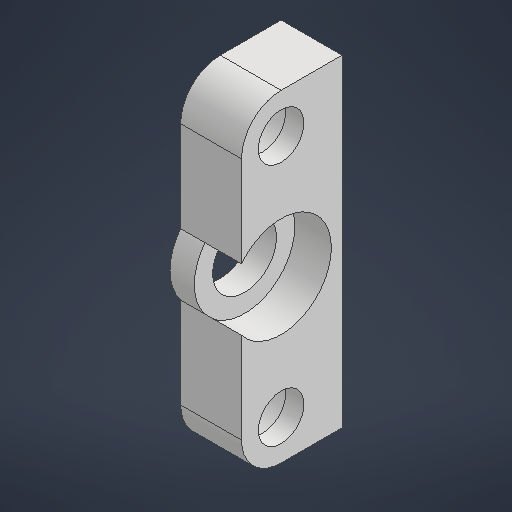
# Autodesk Inventor part: PCB_Housing_07_V4
Saved by Autodesk Inventor 2026.2 (Build 302298000, 298)
## iProperties
Created: 2026-03-17
Part Number: PCB_Housing_07_V4
Material: Generic
Document SubType Name: Modeling
Designer: vckot
Density: 1 g/cm^3
Appearance: Default
Author: vckot
Autodesk Inventor part; units mm, degrees
ref_plane "YZ Plane" through (0, 0, 0) normal (1, 0, 0) x (0, 1, 0)
ref_plane "XZ Plane" through (0, 0, 0) normal (0, 1, 0) x (-1, 0, 0)
ref_plane "XY Plane" through (0, 0, 0) normal (0, 0, 1) x (1, 0, 0)
sketch "Sketch1" plane through (0, 0, 0) normal (1, 0, 0) x (0, 1, 0)
  circle A0 centre (0, 0) radius 4.125
  line L0 (-4.125, 0) -> (-4.125, -5)
  line L1 (4.125, 0) -> (4.125, -5)
  line L2 (-4.125, -5) -> (4.125, -5)
  circle A1 centre (-10, 0) radius 2.25
  circle A2 centre (10, 0) radius 2.25
  circle A3 centre (-10, 0) radius 3.25
  circle A4 centre (10, 0) radius 3.25
  line L3 (-10, 3.25) -> (-2.5403, 3.25)
  line L4 (10, 3.25) -> (2.5403, 3.25)
  line L5 (-13.25, 0) -> (-13.25, -5)
  line L6 (13.25, 0) -> (13.25, -5)
  line L7 (-13.25, -5) -> (13.25, -5)
  dimension "d0" = 8.25
  dimension "d1" = 4.5
  dimension "d2" = 4.5
  dimension "d3" = 10
  dimension "d4" = 10
  dimension "d5" = 6.5
  dimension "d6" = 6.5
  dimension "d7" = 5
  dimension "d8" = 5
  dimension "d9" = 26.5
  dimension "d10" = 5
  constraints: 16 end point, 8 point on circle, 5 centre point, 5 tangent, 4 coincident, 2 horizontal alignment, 2 perpendicular, 2 point on line, 1 horizontal, 1 parallel, 1 vertical
  measures "d0" diameter of A0
  measures "d1" diameter of A1
  measures "d2" diameter of A2
  measures "d3" distance of A0.centre A1.centre
  measures "d4" distance of A0.centre A2.centre
  measures "d5" diameter of A3
  measures "d6" diameter of A4
  measures "d7" distance of L6.start L7.end
  measures "d8" distance of L5.start L7.start
  measures "d9" distance of L7.start L7.end
  measures "d10" distance from line of point (0, 0) L2
extrude "Extrusion1" add sketch "Sketch1" along normal blind 5 contours L1 L2 L0 A0 | A0 L4 A4 L6 L7 L1 | L0 L7 L5 A3 L3 A0 | A4 | A3 | A1 | A2
sketch "Sketch2" plane through (0, 0, 0) normal (-1, 0, 0) x (0, 0, 1)
  circle A0 centre (0, 0) radius 2.625
  arc A1 (3.25, 2.5403) -> (3.25, -2.5403) centre (0, 0) ccw projected
  line L0 (3.25, -2.5403) -> (3.25, 2.5403)
  circle A2 centre (0, 10) radius 2.25 projected
  circle A3 centre (0, -10) radius 2.25 projected
  dimension "d13" = 5.25
  constraints: 2 end point, 1 centre point, 1 coincident, 1 vertical
  measures "d13" diameter of A0
extrude "Extrusion2" add sketch "Sketch1" along normal blind 2 contours A0
extrude "Extrusion3" cut sketch "Sketch2" against normal blind 2 contours A0
hole "Hole1" at (0, 10, 0) at (0, -10, 0) direction (1, 0, 0) diameter 3.75 depth 8 tip angle 118 counterbore diameter 6 counterbore depth 3.5
body "Solid1"
